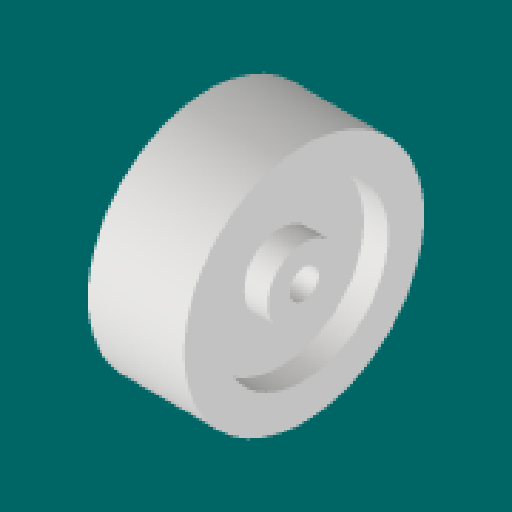
# Autodesk Inventor part: KZ
Saved by Autodesk Inventor 2023 (Build 270158000, 158)
## iProperties
Created: 2023-01-28
Part Number: KZ
Material: Generic
Document SubType Name: Modeling
Designer: HeavyDrewno
Density: 1 g/cm^3
Appearance: Default
Author: HeavyDrewno
Autodesk Inventor part; units mm, degrees
ref_plane "YZ Plane" through (0, 0, 0) normal (1, 0, 0) x (0, 1, 0)
ref_plane "XZ Plane" through (0, 0, 0) normal (0, 1, 0) x (-1, 0, 0)
ref_plane "XY Plane" through (0, 0, 0) normal (0, 0, 1) x (1, 0, 0)
sketch "Sketch1" plane through (0, 0, 0) normal (0, 1, 0) x (-1, 0, 0)
  line L0 (0, 0) -> (0, -6) construction
  line L1 (0, -6) -> (40, -6)
  line L2 (40, -6) -> (40, -50) construction
  line L3 (40, -50) -> (0, -50)
  line L4 (0, -50) -> (0, -35)
  line L5 (0, -35) -> (10, -35)
  line L6 (10, -35) -> (10, -15)
  line L7 (10, -15) -> (0, -15)
  line L8 (0, -15) -> (0, -6)
  line L9 (20, -6) -> (20, -50) construction
  line L10 (40, -50) -> (40, -35)
  line L11 (40, -35) -> (30, -35)
  line L12 (30, -35) -> (30, -15)
  line L13 (30, -15) -> (40, -15)
  line L14 (40, -15) -> (40, -6)
  line L15 (0, 0) -> (40, 0) construction
  dimension "d0" = 6
  dimension "d1" = 40
  dimension "d2" = 44
  dimension "d3" = 15
  dimension "d4" = 10
  dimension "d5" = 20
  constraints: 32 end point, 8 perpendicular, 4 symmetric about line, 2 midpoint, 2 point on line, 1 horizontal, 1 vertical
  measures "d0" distance of L0.start L0.end
  measures "d1" distance of L0.end L1.end
  measures "d2" distance of L1.end L2.end
  measures "d3" distance of L3.end L4.end
  measures "d4" distance of L4.end L5.end
  measures "d5" distance of L5.end L6.end
revolve "Revolution1" add sketch "Sketch1" angle 360 about axis through (0, 0, 0) along (-1, 0, 0)
body "Solid1"
